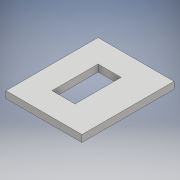
# Autodesk Inventor part: kunci
Saved by Autodesk Inventor 2017 (Build 210142000, 142)
## iProperties
Created: 2017-01-17
Part Number: kunci
Material: Generic
Document SubType Name: Modeling
Designer: Ghesa Bhakti
Density: 1 g/cm^3
Appearance: Default
Author: Ghesa Bhakti
Autodesk Inventor part; units mm, degrees
ref_plane "YZ Plane" through (0, 0, 0) normal (1, 0, 0) x (0, 1, 0)
ref_plane "XZ Plane" through (0, 0, 0) normal (0, 1, 0) x (-1, 0, 0)
ref_plane "XY Plane" through (0, 0, 0) normal (0, 0, 1) x (1, 0, 0)
sketch "Sketch1" plane through (0, 0, 0) normal (0, 0, 1) x (1, 0, 0)
  line L0 (0, 120) -> (-30, 120)
  line L1 (-30, 120) -> (-30, 80)
  line L2 (-30, 80) -> (0, 80)
  line L3 (-20, 110) -> (-10, 110)
  line L4 (-10, 110) -> (-10, 90)
  line L5 (-10, 90) -> (-20, 90)
  line L6 (-20, 90) -> (-20, 110)
  line L7 (0, 120) -> (3, 120)
  line L8 (3, 120) -> (3, 80)
  line L9 (3, 80) -> (0, 80)
  line L10 (-30, 120) -> (3, 120)
  line L11 (3, 120) -> (3, 80)
  line L12 (3, 80) -> (-30, 80)
  line L13 (-30, 80) -> (-30, 120)
  point P0 (0, 0)
  constraints: 28 end point, 6 parallel, 4 horizontal, 4 perpendicular
extrude "Extrusion1" add sketch "Sketch1" along normal blind 3
body "Solid1"
